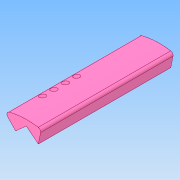
# Autodesk Inventor part: ContactMount
Saved by Autodesk Inventor 2017.3 (Build 213256000, 256)
## iProperties
Created: 2019-06-19
Part Number: ContactMount
Material: ABS Plastic
Document SubType Name: Modeling
Designer: Derek Wider
Density: 1.06 g/cm^3
Appearance: Pink
Author: Derek Wider
Autodesk Inventor part; units mm, degrees
ref_plane "YZ Plane" through (0, 0, 0) normal (1, 0, 0) x (0, 1, 0)
ref_plane "XZ Plane" through (0, 0, 0) normal (0, 1, 0) x (-1, 0, 0)
ref_plane "XY Plane" through (0, 0, 0) normal (0, 0, 1) x (1, 0, 0)
sketch "Sketch1" plane through (0, 0, 0) normal (0, 0, 1) x (1, 0, 0)
  line L0 (0, 0) -> (4.826, 4.3221)
  line L1 (4.826, 4.3221) -> (10.16, 0)
  line L2 (10.16, 0) -> (11.43, 6.2217)
  line L3 (0, 0) -> (-4.975, 5.229)
  arc A0 (11.43, 6.2217) -> (-4.975, 5.229) centre (5.08, -24.8868) ccw
  circle A1 centre (5.08, -24.8868) radius 25.4 construction
  dimension "d0" = 31.75
  dimension "d2" = 50.8
  dimension "d3" = 29.21
  dimension "d4" = 30
  dimension "d5" = 10.16
  dimension "d6" = 5.334
  constraints: 8 end point, 4 point on circle, 2 centre point, 1 coincident, 1 horizontal alignment, 1 line through centre
  measures "d0" radius of A0
  measures "d2" diameter of A1
  measures "d3" distance of A1.centre L0.end
  measures "d5" distance of L1.end L0.start
  measures "d6" horizontal distance of L1.end L0.end
extrude "Extrusion1" add sketch "Sketch1" along normal blind 59.2074
fillet "Fillet1" radius 1.27 2 edges at (-4.975, 5.229, 29.6037) (11.43, 6.2217, 29.6037)
sketch "Sketch2" plane through (4.826, 4.3221, 0) normal (0.6671445, -0.7449283, 0) x (0.7449283, 0.6671445, 0)
  line L0 (-6.4785, 59.2074) -> (0, 59.2074) construction
  circle A0 centre (-3.3035, 45.8724) radius 1.27
  line L1 (-6.4785, 0) -> (-6.4785, 59.2074) projected
  dimension "d10" = 13.335
  dimension "d11" = 3.175
  dimension "d12" = 2.54
  constraints: 1 centre point
  measures "d10" distance from line of A0.centre L0
  measures "d11" distance from line of L1 A0.centre
  measures "d12" diameter of A0
extrude "Extrusion2" cut sketch "Sketch2" against normal through all
pattern_linear "Rectangular Pattern1" count 4 spacing 5.08 along (0, 0, -1) of "Extrusion2"
sketch "Sketch3" plane through (4.826, 4.3221, 0) normal (0.6671445, -0.7449283, 0) x (0.7449283, 0.6671445, 0)
  circle A0 centre (-3.3035, 30.6324) radius 1.27 construction
  circle A1 centre (-3.3035, 35.7124) radius 1.27 construction
  circle A2 centre (-3.3035, 40.7924) radius 1.27 construction
  circle A3 centre (-3.3035, 45.8724) radius 1.27 construction
  line L0 (-6.4785, 0) -> (0, 0) construction
  line L1 (0, 0) -> (0, 59.2074) construction
  line L2 (-6.4785, 59.2074) -> (0, 59.2074) construction
  line L3 (-6.4785, 0) -> (-6.4785, 59.2074) construction
  line L4 (-6.4785, 0) -> (-6.4785, 59.2074) projected
  line L5 (0, 0) -> (0, 59.2074) projected
  line L6 (-6.4785, 48.1584) -> (0, 48.1584)
  line L7 (0, 48.1584) -> (0, 48.6664)
  line L8 (0, 48.6664) -> (-6.4785, 48.6664)
  line L9 (-6.4785, 48.6664) -> (-6.4785, 48.1584)
  dimension "d18" = 2.286
  dimension "d19" = 0.508
  constraints: 8 end point, 2 parallel, 2 point on line, 1 horizontal, 1 perpendicular
  measures "d18" distance from line of L6 A3.centre
  measures "d19" distance between parallel lines of L6 L8
extrude "Extrusion3" add sketch "Sketch3" along normal blind 1.524
chamfer "Chamfer1" distance 0.762 angle 45 2 edges at (2.413, 2.161, 48.6664) (2.413, 2.161, 48.1584)
pattern_linear "Rectangular Pattern3" count 5 spacing 5.08 along (0, 0, -1) of "Extrusion3", "Chamfer1"
body "Solid1"
